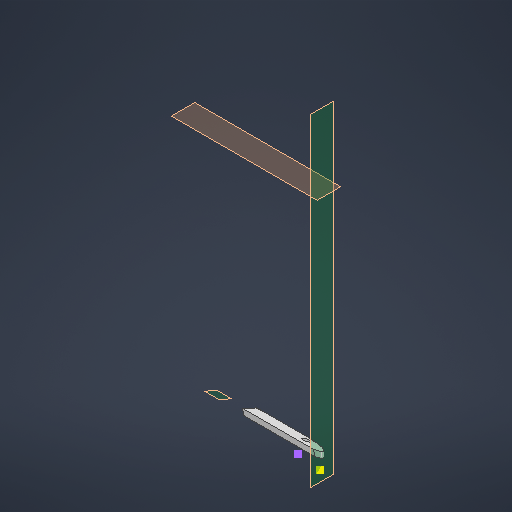
# Autodesk Inventor part: connector
Saved by Autodesk Inventor 2026 (Build 300175050, 175E)
## iProperties
Created: 2026-06-09
Part Number: connector
Material: Generic
Document SubType Name: Modeling
Designer: Delbe
Density: 1 g/cm^3
Appearance: Default
Author: Delbe
Autodesk Inventor part; units mm, degrees
sketch "Sketch5" plane through (0, 0, 0) normal (0, 1, 0) x (-1, 0, 0)
  spline S0 degree 4 poles (214, 0.3449) (213.9235, 0.3586) (213.5504, 0.4255) (212.9247, 0.5375) (211.8694, 0.7251) (210.7617, 0.9209) (209.4043, 1.1592) (207.8102, 1.4368) (205.9789, 1.7525) (203.9169, 2.1042) (201.6282, 2.4897) (199.1185, 2.907) (196.3936, 3.3535) (193.4599, 3.8269) (190.3242, 4.3245) (186.9939, 4.8439) (183.4768, 5.3823) (179.781, 5.937) (175.9152, 6.5054) (171.8885, 7.0847) (167.7102, 7.6721) (163.3902, 8.265) (158.9384, 8.8603) (154.3653, 9.4553) (149.6816, 10.047) (144.8982, 10.6323) (140.0263, 11.2083) (135.0773, 11.7717) (130.0627, 12.3193) (124.9942, 12.8478) (119.8837, 13.3538) (114.7431, 13.8337) (109.5844, 14.2841) (104.4196, 14.7015) (99.2609, 15.0822) (94.1202, 15.4227) (89.0095, 15.7197) (83.9407, 15.9697) (78.9258, 16.1695) (73.9764, 16.3162) (69.104, 16.4071) (64.32, 16.4396) (59.6357, 16.4118) (55.0618, 16.3218) (50.6091, 16.1683) (46.288, 15.9504) (42.1085, 15.6678) (38.0804, 15.3204) (34.213, 14.9088) (30.5154, 14.4338) (26.9962, 13.8969) (23.6634, 13.3) (20.5248, 12.6451) (17.5876, 11.9348) (14.8584, 11.1717) (12.3433, 10.3589) (10.0479, 9.4991) (7.977, 8.5956) (6.1348, 7.651) (4.5247, 6.6676) (3.1496, 5.6471) (2.0123, 4.5896) (1.1163, 3.495) (0.468, 2.3618) (0.0758, 1.1958) (-0.0534, 0) (0.0758, -1.1958) (0.468, -2.3618) (1.1163, -3.495) (2.0123, -4.5896) (3.1496, -5.6471) (4.5247, -6.6676) (6.1348, -7.651) (7.977, -8.5956) (10.0479, -9.4991) (12.3433, -10.3589) (14.8584, -11.1717) (17.5876, -11.9348) (20.5248, -12.6451) (23.6634, -13.3) (26.9962, -13.8969) (30.5154, -14.4338) (34.213, -14.9088) (38.0804, -15.3204) (42.1085, -15.6678) (46.288, -15.9504) (50.6091, -16.1683) (55.0618, -16.3218) (59.6357, -16.4118) (64.32, -16.4396) (69.104, -16.4071) (73.9764, -16.3162) (78.9258, -16.1695) (83.9407, -15.9697) (89.0095, -15.7197) (94.1202, -15.4227) (99.2609, -15.0822) (104.4196, -14.7015) (109.5844, -14.2841) (114.7431, -13.8337) (119.8837, -13.3538) (124.9942, -12.8478) (130.0627, -12.3193) (135.0773, -11.7717) (140.0263, -11.2083) (144.8982, -10.6323) (149.6816, -10.047) (154.3653, -9.4553) (158.9384, -8.8603) (163.3902, -8.265) (167.7102, -7.6721) (171.8885, -7.0847) (175.9152, -6.5054) (179.781, -5.937) (183.4768, -5.3823) (186.9939, -4.8439) (190.3242, -4.3245) (193.4599, -3.8269) (196.3936, -3.3535) (199.1185, -2.907) (201.6282, -2.4897) (203.9169, -2.1042) (205.9789, -1.7525) (207.8102, -1.4368) (209.4043, -1.1592) (210.7617, -0.9209) (211.8694, -0.7251) (212.9247, -0.5375) (213.5504, -0.4255) (213.9235, -0.3586) (214, -0.3449) knots 0 0 0 0 0 0.006275 0.009968 0.014263 0.019074 0.024344 0.030027 0.036088 0.042498 0.04923 0.056263 0.063574 0.071147 0.078961 0.087003 0.095255 0.103702 0.112331 0.121128 0.130079 0.13917 0.148391 0.157726 0.167166 0.176696 0.186306 0.195983 0.205715 0.215491 0.225299 0.235127 0.244964 0.254798 0.264619 0.274414 0.284172 0.293881 0.303532 0.313111 0.322608 0.332012 0.34131 0.350493 0.359549 0.368466 0.377233 0.385838 0.39427 0.402518 0.410569 0.418411 0.426034 0.433424 0.440569 0.447459 0.454083 0.460432 0.466498 0.472281 0.477786 0.483031 0.48805 0.4929 0.497646 0.502354 0.5071 0.51195 0.516969 0.522214 0.527719 0.533502 0.539568 0.545917 0.552541 0.559431 0.566576 0.573966 0.581589 0.589431 0.597482 0.60573 0.614162 0.622767 0.631534 0.640451 0.649507 0.65869 0.667988 0.677392 0.686889 0.696468 0.706119 0.715828 0.725586 0.735381 0.745202 0.755036 0.764873 0.774701 0.784509 0.794285 0.804017 0.813694 0.823304 0.832834 0.842274 0.851609 0.86083 0.869921 0.878872 0.887669 0.896298 0.904745 0.912997 0.921039 0.928853 0.936426 0.943737 0.95077 0.957502 0.963912 0.969973 0.975656 0.980926 0.985737 0.990032 0.993725 1 1 1 1 1
  line L0 (204.525, -2) -> (204.525, 2)
  line L1 (204.525, 0) -> (0, 0)
  line L2 (0, 0) -> (61.2, 0)
  line L3 (61.2, 0) -> (61.2, -16.415)
  line L4 (61.2, -16.415) -> (61.2, 16.415)
  point P0 (0, 0)
  point P1 (213.875, 0.3673)
  point P2 (213.5005, 0.4344)
  point P3 (212.8772, 0.5457)
  point P4 (212.0066, 0.7006)
  point P5 (210.8908, 0.8979)
  point P6 (209.5323, 1.1364)
  point P7 (207.9344, 1.4146)
  point P8 (206.1007, 1.7309)
  point P9 (204.0356, 2.0831)
  point P10 (201.7438, 2.4693)
  point P11 (199.2308, 2.8872)
  point P12 (196.5023, 3.3344)
  point P13 (193.5648, 3.8084)
  point P14 (190.4252, 4.3068)
  point P15 (187.0907, 4.8269)
  point P16 (183.5691, 5.366)
  point P17 (179.8687, 5.9215)
  point P18 (175.9981, 6.4907)
  point P19 (171.9664, 7.0708)
  point P20 (167.7829, 7.6591)
  point P21 (163.4575, 8.2526)
  point P22 (159.0002, 8.8488)
  point P23 (154.4215, 9.4444)
  point P24 (149.732, 10.0368)
  point P25 (144.9427, 10.6228)
  point P26 (140.0648, 11.1993)
  point P27 (135.1097, 11.7633)
  point P28 (130.0889, 12.3114)
  point P29 (125.0142, 12.8402)
  point P30 (119.8974, 13.3464)
  point P31 (114.7505, 13.8266)
  point P32 (109.5855, 14.2771)
  point P33 (104.4145, 14.6943)
  point P34 (99.2495, 15.0749)
  point P35 (94.1026, 15.4151)
  point P36 (88.9858, 15.7116)
  point P37 (83.9111, 15.961)
  point P38 (78.8903, 16.1601)
  point P39 (73.9352, 16.306)
  point P40 (69.0573, 16.3958)
  point P41 (64.268, 16.4271)
  point P42 (59.5785, 16.3978)
  point P43 (54.9998, 16.3062)
  point P44 (50.5425, 16.1509)
  point P45 (46.2171, 15.931)
  point P46 (42.0336, 15.6461)
  point P47 (38.0019, 15.2962)
  point P48 (34.1313, 14.8818)
  point P49 (30.4309, 14.4038)
  point P50 (26.9093, 13.8636)
  point P51 (23.5748, 13.2629)
  point P52 (20.4352, 12.6039)
  point P53 (17.4977, 11.889)
  point P54 (14.7693, 11.1209)
  point P55 (12.2562, 10.3027)
  point P56 (9.9644, 9.4372)
  point P57 (7.8993, 8.5276)
  point P58 (6.0656, 7.5769)
  point P59 (4.4677, 6.5883)
  point P60 (3.1092, 5.5644)
  point P61 (1.9934, 4.5081)
  point P62 (1.1228, 3.4216)
  point P63 (0.4995, 2.307)
  point P64 (0.125, 1.1661)
  point P65 (0.125, -1.1661)
  point P66 (0.4995, -2.307)
  point P67 (1.1228, -3.4216)
  point P68 (1.9934, -4.5081)
  point P69 (3.1092, -5.5644)
  point P70 (4.4677, -6.5883)
  point P71 (6.0656, -7.5769)
  point P72 (7.8993, -8.5276)
  point P73 (9.9644, -9.4372)
  point P74 (12.2562, -10.3027)
  point P75 (14.7693, -11.1209)
  point P76 (17.4977, -11.889)
  point P77 (20.4352, -12.6039)
  point P78 (23.5748, -13.2629)
  point P79 (26.9093, -13.8636)
  point P80 (30.4309, -14.4038)
  point P81 (34.1313, -14.8818)
  point P82 (38.0019, -15.2962)
  point P83 (42.0336, -15.6461)
  point P84 (46.2171, -15.931)
  point P85 (50.5425, -16.1509)
  point P86 (54.9998, -16.3062)
  point P87 (59.5785, -16.3978)
  point P88 (64.268, -16.4271)
  point P89 (69.0573, -16.3958)
  point P90 (73.9352, -16.306)
  point P91 (78.8903, -16.1601)
  point P92 (83.9111, -15.961)
  point P93 (88.9858, -15.7116)
  point P94 (94.1026, -15.4151)
  point P95 (99.2495, -15.0749)
  point P96 (104.4145, -14.6943)
  point P97 (109.5855, -14.2771)
  point P98 (114.7505, -13.8266)
  point P99 (119.8974, -13.3464)
  point P100 (125.0142, -12.8402)
  point P101 (130.0889, -12.3114)
  point P102 (135.1097, -11.7633)
  point P103 (140.0648, -11.1993)
  point P104 (144.9427, -10.6228)
  point P105 (149.732, -10.0368)
  point P106 (154.4215, -9.4444)
  point P107 (159.0002, -8.8488)
  point P108 (163.4575, -8.2526)
  point P109 (167.7829, -7.6591)
  point P110 (171.9664, -7.0708)
  point P111 (175.9981, -6.4907)
  point P112 (179.8687, -5.9215)
  point P113 (183.5691, -5.366)
  point P114 (187.0907, -4.8269)
  point P115 (190.4252, -4.3068)
  point P116 (193.5648, -3.8084)
  point P117 (196.5023, -3.3344)
  point P118 (199.2308, -2.8872)
  point P119 (201.7438, -2.4693)
  point P120 (204.0356, -2.0831)
  point P121 (206.1007, -1.7309)
  point P122 (207.9344, -1.4146)
  point P123 (209.5323, -1.1364)
  point P124 (210.8908, -0.8979)
  point P125 (212.0066, -0.7006)
  point P126 (212.8772, -0.5457)
  point P127 (213.5005, -0.4344)
  point P128 (213.875, -0.3673)
  dimension "d28" = 204.525
  dimension "d29" = 61.2
  dimension "d30" = 32.8299
  constraints: 10 end point, 2 point on line, 1 horizontal, 1 midpoint, 1 perpendicular, 1 vertical, 135 other
  measures "d28" distance of L1.start L1.end
  measures "d29" distance of L1.end L2.end
  measures "d30" distance of L3.end L4.end
extrude "Main Wing" add sketch "Sketch5" along normal blind 453.491
sketch "Sketch6" plane through (-204.525, 0, 2) normal (-1, 0, 0) x (0, 0, 1)
  line L0 (0, 0) -> (0, 66.548)
  line L1 (0, 453.4889) -> (0, 366.5701)
  line L2 (20, 366.5701) -> (-20, 366.5701)
  line L3 (-20, 66.548) -> (20, 66.548)
  line L4 (20, 66.548) -> (20, 366.5701)
  line L5 (-20, 366.5701) -> (-20, 66.548)
  point P0 (-2, 0)
  dimension "d31" = 66.548
  dimension "d32" = 86.9188
  dimension "d33" = 40
  dimension "d34" = 40
  dimension "d43" = 300.0221
  constraints: 12 end point, 3 vertical, 2 horizontal, 2 midpoint
  measures "d31" distance of L0.start L0.end
  measures "d32" distance of L1.start L1.end
  measures "d33" distance of L2.start L2.end
  measures "d34" distance of L3.start L3.end
  measures "d43" distance of L3.end L2.start
extrude "Rectangle Elevron Gap" cut sketch "Sketch6" against normal blind 69.6214
sketch "Sketch7" plane through (-204.525, 66.548, 2) normal (0, 1, 0) x (1, 0, 0)
  line L0 (69.6201, 13.7865) -> (69.6201, -9.7851)
  line L1 (69.6201, -9.7851) -> (69.6201, 2.0009)
  circle A0 centre (69.6201, 2.0009) radius 17
  circle A1 centre (69.6201, 2.0009) radius 1.7526
  point P0 (204.525, 2)
  point P1 (69.6201, 3.7535)
  point P2 (69.6201, 0.2483)
  dimension "d37" = 23.5717
  dimension "d38" = 11.786
  dimension "d41" = 34
  dimension "d42" = 3.5052
  constraints: 4 end point, 2 centre point, 1 coincident, 1 point on line, 1 vertical
  measures "d37" distance of L0.start L0.end
  measures "d38" distance of L0.end L1.end
  measures "d41" diameter of A0
  measures "d42" diameter of A1
extrude "Circle Elevron Gap" cut sketch "Sketch7" along normal blind 300.0221 contours A1 L0 | A0 picked at (69.7501, 0.8471)
sketch "Sketch8" plane through (0, 453.491, 0) normal (0, 1, 0) x (1, 0, 0)
  line L0 (-204.5238, 0) -> (-143.0304, 0)
  circle A0 centre (-143.0304, 0) radius 1.7526
  point P0 (0, 0)
  dimension "d46" = 61.4934
  dimension "d47" = 3.5052
  constraints: 2 end point, 1 centre point, 1 coincident, 1 horizontal
  measures "d46" distance of L0.start L0.end
  measures "d47" diameter of A0
extrude "Elevron Screw Hole" cut sketch "Sketch8" against normal blind 454.0221
ref_plane "Leading Edge Plane" through (0, 226.7455, 0) normal (-1, 0, 0) x (0, 0, 1)
sketch "Sketch9" plane through (0, 226.7455, 0) normal (-1, 0, 0) x (0, 0, 1)
  line L0 (0, -226.7455) -> (0, 226.7401)
  line L1 (0, 226.7401) -> (0, 213.1781)
  line L2 (0, 213.1781) -> (0, 194.4281)
  circle A0 centre (0, 194.4281) radius 18.75
  line L3 (-14.0018, 198.1799) -> (3.7518, 208.4299)
  line L4 (3.7518, 208.4299) -> (14.0018, 190.6764)
  line L5 (14.0018, 190.6764) -> (-3.7518, 180.4264)
  line L6 (-3.7518, 180.4264) -> (-14.0018, 198.1799)
  line L7 (-14.0018, 198.1799) -> (14.0018, 190.6764) construction
  line L8 (3.7518, 208.4299) -> (-3.7518, 180.4264) construction
  circle A1 centre (0, 194.4281) radius 15.5
  dimension "d50" = 13.562
  dimension "d51" = 18.75
  dimension "d52" = 37.5
  dimension "d55" = 20.5
  dimension "d56" = 20.5
  dimension "d70" = 31
  constraints: 18 end point, 2 centre point, 2 coincident, 2 midpoint, 2 parallel, 2 point on line, 1 perpendicular, 1 vertical
  measures "d50" distance of L0.end L1.end
  measures "d51" distance of L1.end L2.end
  measures "d52" diameter of A0
  measures "d55" distance of L4.end L5.end
  measures "d56" distance of L3.end L4.end
  measures "d70" diameter of A1
extrude "Circle thingy for boom" add sketch "Sketch9" along normal blind 204.5 contours A1 L0 L3 L6 L5 | L0 L5 L4 L3 A1 | L5 L6 L3 L0 | L0 L3 L4 L5
sketch "Sketch10" plane through (0, 226.7455, 0) normal (1, 0, 0) x (0, 0, -1)
  line L0 (0, 213.1791) -> (0, 194.4291)
  line L1 (13.6215, 199.3869) -> (-4.9578, 208.0506)
  line L2 (-4.9578, 208.0506) -> (-13.6215, 189.4713)
  line L3 (-13.6215, 189.4713) -> (4.9578, 180.8076)
  line L4 (4.9578, 180.8076) -> (13.6215, 199.3869)
  line L5 (13.6215, 199.3869) -> (-13.6215, 189.4713) construction
  line L6 (-4.9578, 208.0506) -> (4.9578, 180.8076) construction
  point P0 (0, -226.7455)
  dimension "d57" = 18.75
  dimension "d58" = 20.5
  dimension "d59" = 20.5
  constraints: 14 end point, 2 parallel, 1 perpendicular, 1 vertical
  measures "d57" distance of L0.start L0.end
  measures "d58" distance of L3.end L2.end
  measures "d59" distance of L2.end L1.end
extrude "20x20 hole for boom" cut sketch "Sketch10" against normal blind 205.5
ref_plane "Plane of Pain" through (-204.525, 0, -17) normal (0, 0, 1) x (0, 1, 0)
ref_plane "Work Plane5" through (-204.525, 0, -2) normal (0, 0, 1) x (0, 1, 0)
sketch "Sketch11" plane through (-204.525, 0, -17) normal (0, 0, 1) x (0, 1, 0)
  line L0 (453.4842, 0.0013) -> (403.4842, 0.0013)
  line L1 (403.4842, 0.0013) -> (404.7122, -149.9936)
  circle A0 centre (404.7122, -149.9936) radius 5.25
  line L2 (404.7122, -149.9936) -> (219.7122, -149.9936)
  circle A1 centre (219.7122, -149.9936) radius 5.25
  line L3 (366.5707, -80.63) -> (219.7122, -80.63)
  line L4 (219.7122, -80.63) -> (219.7122, -149.9936)
  point P0 (0, -204.525)
  dimension "d64" = 50
  dimension "d65" = 150
  dimension "d66" = 10.5
  dimension "d67" = 185
  dimension "d121" = 146.8585
  dimension "d122" = 69.3637
  constraints: 10 end point, 3 horizontal, 2 centre point, 2 coincident, 1 equal radius, 1 perpendicular
  measures "d64" distance of L0.start L0.end
  measures "d65" distance of L0.end L1.end
  measures "d66" diameter of A0
  measures "d67" distance of L2.start L2.end
  measures "d121" distance of L3.start L3.end
  measures "d122" distance of L3.end L4.end
ref_plane "20x20 Plane" through (0, 416.8428, -9.2897) normal (0, 0.4226183, 0.9063078) x (1, 0, 0)
sketch "Sketch12" plane through (0, 416.8428, -9.2897) normal (0, 0.4226183, 0.9063078) x (1, 0, 0)
  line L0 (0, 10.2503) -> (0, 0.0003)
  line L1 (0, 0.0003) -> (-55, 0.0003)
  circle A0 centre (-55, 0.0003) radius 5.25
  circle A1 centre (-55, 0.0003) radius 2.75
  point P0 (0, -381.7138)
  dimension "d71" = 10.25
  dimension "d72" = 55
  dimension "d73" = 10.5
  dimension "d74" = 5.5
  constraints: 4 end point, 3 coincident, 2 centre point, 1 horizontal, 1 vertical
  measures "d71" distance of L0.start L0.end
  measures "d72" distance of L0.end L1.end
  measures "d73" diameter of A0
  measures "d74" diameter of A1
sketch "Sketch13" plane through (0, 416.8428, -9.2897) normal (0, 0.4226183, 0.9063078) x (1, 0, 0)
  circle A0 centre (-55, 0) radius 5.25
  circle A1 centre (-55, 0) radius 2.75
  point P0 (0, -381.7138)
  dimension "d77" = 10.5
  dimension "d82" = 5.5
  constraints: 2 centre point, 1 coincident
  measures "d77" diameter of A0
  measures "d82" diameter of A1
extrude "Boom Screw Head" cut sketch "Sketch13" against normal blind 13.75 contours A0 | A1
extrude "Boom Screw Hole" add sketch "Sketch12" against normal blind 3
sketch "Sketch14" plane through (-204.525, 366.5701, -2) normal (0, -1, 0) x (1, 0, 0)
  line L0 (61.5404, 3.7631) -> (61.5404, 7.2141)
  line L1 (61.5404, 7.2141) -> (43.5474, 7.2141)
  line L2 (61.5404, 7.2141) -> (69.3184, 7.2141)
  line L3 (43.5474, 7.2141) -> (43.5474, -10.2859)
  line L4 (69.3184, 7.2141) -> (69.3184, -10.2859)
  line L5 (43.5474, -10.2859) -> (69.3184, -10.2859)
  point P0 (204.525, 2)
  dimension "d89" = 3.451
  dimension "d90" = 17.993
  dimension "d91" = 7.778
  dimension "d93" = 17.5
  dimension "d94" = 17.5
  constraints: 12 end point, 3 vertical, 2 horizontal
  measures "d89" distance of L0.start L0.end
  measures "d90" distance of L0.end L1.end
  measures "d91" distance of L0.end L2.end
  measures "d93" distance of L1.end L3.end
  measures "d94" distance of L2.end L4.end
extrude "Servo Hole" cut sketch "Sketch14" against normal blind 28.763
sketch "Sketch15" plane through (-135.2066, 366.5701, -11.7525) normal (-1, 0, 0) x (0, 0, 1)
  line L0 (17, 0) -> (17, 6)
  line L1 (17, 6) -> (17, 8)
  line L2 (17, 8) -> (-3, 8)
  line L3 (-3, 8) -> (-3, 6)
  line L4 (-3, 6) -> (17, 6)
  point P0 (11.7525, -366.5701)
  dimension "d97" = 6
  dimension "d98" = 2
  dimension "d99" = 2
  constraints: 10 end point, 2 perpendicular, 1 point on line, 1 vertical
  measures "d97" distance of L0.start L0.end
  measures "d98" distance of L0.end L1.end
  measures "d99" distance of L2.end L3.end
extrude "Servo Sidewall 1" cut sketch "Sketch15" against normal blind 2.782
sketch "Sketch16" plane through (-160.9776, 366.5701, 5.2141) normal (1, 0, 0) x (0, 0, -1)
  line L0 (0, 0) -> (0, 6)
  line L1 (0, 6) -> (0, 8)
  line L2 (0, 8) -> (14, 8)
  line L3 (14, 8) -> (14, 6)
  line L4 (14, 6) -> (0, 6)
  point P0 (5.2141, -366.5701)
  dimension "d102" = 6
  dimension "d103" = 2
  constraints: 10 end point, 2 perpendicular, 1 point on line, 1 vertical
  measures "d102" distance of L0.start L0.end
  measures "d103" distance of L0.end L1.end
extrude "Servo Sidewall 2" cut sketch "Sketch16" against normal blind 2.782
sketch "Sketch17" plane through (-135.2066, 366.5701, 5.2141) normal (0, 0, -1) x (-1, 0, 0)
  line L0 (0, 8) -> (0, 16.3)
  line L1 (0, 28.7478) -> (0, 23.2698)
  line L2 (0, 16.3) -> (-27.1565, 48.6638)
  line L3 (0, 23.2698) -> (-27.1565, 55.6336)
  line L4 (-27.1565, 48.6638) -> (-27.1565, 55.6336)
  line L5 (0, 23.2698) -> (0, 16.3)
  point P0 (-135.2066, -366.5701)
  point P1 (0, 23.2698)
  dimension "d106" = 8.3
  dimension "d107" = 5.478
  dimension "d108" = 42.248
  dimension "d109" = 42.248
  constraints: 12 end point, 3 vertical, 1 coincident, 1 point on line
  measures "d106" distance of L0.end L0.start
  measures "d107" distance of L1.end L1.start
  measures "d108" distance of L2.start L2.end
  measures "d109" distance of L3.start L3.end
extrude "some slant hole" cut sketch "Sketch17" along normal blind 23.75
fillet "Fillet for slant" radius 7.7 2 edges at (-135.2066, 382.8701, -3.2692) (-135.2066, 389.8399, -3.2692)
sketch "Sketch18" plane through (-204.525, 0, -17) normal (0, 0, 1) x (0, 1, 0)
  circle A0 centre (219.7124, -149.9979) radius 3.25
  point P0 (0, -204.525)
  dimension "d113" = 6.5
  constraints: 1 centre point
  measures "d113" diameter of A0
extrude "Screwhead for something" cut sketch "Sketch11" along normal blind 5.25 contours A1 L4 L2 | L2 L4 A1
extrude "screwhole for thingy" cut sketch "Sketch18" along normal blind 41.75
ref_plane "Work Plane10" through (-182.7513, 87.2769, 166.4641) normal (0, 0.8660254, -0.5) x (1, 0, 0)
ref_plane "Work Plane9" through (-182.7513, 366.5701, 5.2141) normal (0, 0.8660254, -0.5) x (1, 0, 0)
sketch "Sketch20" plane through (-182.7513, 87.2769, 166.4641) normal (0, 0.8660254, -0.5) x (1, 0, 0)
  circle A0 centre (138, 200) radius 2.8284
  point P0 (182.7513, 187.8006)
  constraints: 1 centre point
ref_plane "Bottom of Airfoil" through (-204.525, 0, 16.5) normal (0, 0, 1) x (0, 1, 0)
sketch "Sketch21" plane through (-204.525, 0, 16.5) normal (0, 0, 1) x (0, 1, 0)
  line L0 (366.5707, -80.6294) -> (219.7127, -80.6294)
  line L1 (219.7127, -80.6294) -> (219.7127, -149.9934)
  line L2 (219.7127, -149.9934) -> (214.6627, -149.9934)
  line L3 (214.6627, -147.0779) -> (214.6627, -152.9089)
  line L4 (214.6627, -147.0779) -> (219.7125, -144.1624)
  line L5 (219.7125, -144.1624) -> (224.7623, -147.0779)
  line L6 (224.7623, -147.0779) -> (224.7623, -152.9089)
  line L7 (224.7623, -152.9089) -> (219.7125, -155.8244)
  line L8 (214.6627, -152.9089) -> (219.7125, -155.8244)
  point P0 (0, -204.525)
  point P1 (224.7623, -147.0779)
  dimension "d123" = 146.858
  dimension "d124" = 69.364
  dimension "d125" = 5.05
  dimension "d126" = 5.831
  dimension "d127" = 5.831
  dimension "d128" = 5.831
  dimension "d129" = 5.831
  dimension "d130" = 5.831
  constraints: 18 end point, 2 perpendicular, 1 horizontal, 1 midpoint, 1 vertical
  measures "d123" distance of L0.start L0.end
  measures "d124" distance of L0.end L1.end
  measures "d125" distance of L1.end L2.end
  measures "d126" distance of L3.start L3.end
  measures "d127" distance of L4.end L4.start
  measures "d128" distance of L5.end L5.start
  measures "d129" distance of L6.end L6.start
  measures "d130" distance of L7.start L7.end
extrude "Hexagon Hole of Doom" cut sketch "Sketch21" against normal blind 4
sketch "Sketch22" plane through (-182.7513, 87.2769, 166.4641) normal (0, 0.8660254, -0.5) x (1, 0, 0)
  line L0 (138, 200) -> (153, 200)
  line L1 (153, 200) -> (153, 185)
  circle A0 centre (153, 185) radius 5.25
  line L2 (153, 185) -> (61.5, 185)
  circle A1 centre (61.5, 185) radius 5.25
  point P0 (182.7513, 187.8006)
  dimension "d137" = 15
  dimension "d138" = 15
  dimension "d139" = 10.5
  dimension "d140" = 91.5
  dimension "d141" = 10.5
  constraints: 6 end point, 2 centre point, 2 coincident, 2 horizontal, 1 vertical
  measures "d137" distance of L0.start L0.end
  measures "d138" distance of L0.end L1.end
  measures "d139" diameter of A0
  measures "d140" distance of L2.start L2.end
  measures "d141" diameter of A1
extrude "Extrusion23" cut sketch "Sketch22" along normal blind 68.25
sketch "Sketch23" plane through (-182.7513, 87.2769, 166.4641) normal (0, 0.8660254, -0.5) x (1, 0, 0)
  line L0 (138, 200) -> (153, 200)
  line L1 (153, 200) -> (153, 185)
  line L2 (153, 185) -> (61.5, 185)
  circle A0 centre (153, 185) radius 5.25
  circle A1 centre (153, 185) radius 3.25
  circle A2 centre (61.5, 185) radius 5.25
  circle A3 centre (61.5, 185) radius 3.25
  point P0 (182.7513, 187.8006)
  dimension "d144" = 15
  dimension "d145" = 15
  dimension "d146" = 91.5
  dimension "d147" = 10.5
  dimension "d148" = 6.5
  dimension "d149" = 10.5
  dimension "d150" = 6.5
  constraints: 6 end point, 4 centre point, 4 coincident, 2 perpendicular, 1 horizontal
  measures "d144" distance of L0.start L0.end
  measures "d145" distance of L0.end L1.end
  measures "d146" distance of L1.end L2.end
  measures "d147" diameter of A0
  measures "d148" diameter of A1
  measures "d149" diameter of A2
  measures "d150" diameter of A3
extrude "Extrusion24" add sketch "Sketch23" along normal blind 20 contours A0 L2 A1 L1 | L1 A1 L2 A0 | A2
sketch "Sketch24" plane through (0, 0, 0) normal (0, -1, 0) x (1, 0, 0)
  line L0 (0, -15) -> (-205, -15)
  line L1 (-205, -15) -> (-205, 16)
  line L2 (-205, 16) -> (0, 16)
  line L3 (0, 16) -> (0, -15)
  point P0 (0, 0)
  constraints: 8 end point, 2 parallel, 1 horizontal, 1 perpendicular
extrude "Extrusion25" cut sketch "Sketch24" along normal blind 8.75
sketch "Sketch25" plane through (0, 226.7455, 0) normal (-1, 0, 0) x (0, 0, 1)
  line L0 (-16.4393, -226.7455) -> (20.5607, -226.7455) construction
  line L1 (17.0941, -211.1086) -> (17.0941, -226.7455)
  line L2 (17.0941, -226.7455) -> (-16.4393, -226.7455)
  line L3 (-16.4393, -226.7455) -> (36.2607, -226.7455) construction
  line L4 (-16.4393, -226.7455) -> (17.4356, -226.7455)
  line L5 (0, -226.7455) -> (0, -219.0797)
  line L6 (17.0941, -201.9506) -> (17.0941, -211.1086)
  line L7 (-36.0788, -226.7455) -> (-16.4393, -226.7455)
  line L8 (-6.752, -213.0525) -> (6.5452, -213.0525) construction
  line L9 (-6.752, -222.2282) -> (6.752, -215.9312)
  line L10 (6.752, -215.9312) -> (7.5873, -206.3837)
  line L11 (7.5873, -206.3837) -> (-14.6028, -216.7311)
  line L12 (-14.6028, -216.7311) -> (-6.752, -222.2282)
  line L13 (-16.4393, -226.7455) -> (17.0941, -211.1086)
  line L14 (17.0941, -226.7455) -> (-16.4393, -226.7455)
  line L15 (-16.4393, -226.7455) -> (-16.4393, 228)
  line L16 (-16.4393, 228) -> (17.0941, 228)
  line L17 (17.0941, 228) -> (17.0941, -226.7455)
  dimension "d155" = 37
  dimension "d220" = 14.9
  dimension "d221" = 60
  dimension "d222" = 60
  dimension "d223" = 8.3
  constraints: 36 end point, 5 horizontal, 3 parallel, 3 vertical, 2 perpendicular, 1 collinear, 1 midpoint, 1 point on line
  measures "d155" distance of L0.start L1.start
  measures "d220" distance of L9.start L9.end
  measures "d221" angle of L10 L11
  measures "d222" angle of L12 L11
  measures "d223" distance between parallel lines of L9 L11
ref_plane "Work Plane14" through (0, 366.491, 0) normal (0, 1, 0) x (1, 0, 0)
ref_plane "Work Plane15" through (-168.2987, 4.1455, -7.5873) normal (0, -0.9063078, 0.4226183) x (1, 0, 0)
extrude "Extrusion36" cut sketch "Sketch25" along normal blind 236.5 contours L13 L10 L11 L12 L15 L16 L17 L6 | L1 L2 L5 L9 L13 | L2 L13 L9 L5
sketch "Sketch35" plane through (-174.1935, 4.5173, -6.752) normal (0, -0.9063078, 0.4226183) x (1, 0, 0)
  line L0 (174.1935, 4.2103) -> (59.1935, 4.2103)
  line L1 (59.1935, 4.2103) -> (59.1935, 22)
  line L2 (59.1935, 22) -> (-35, 22)
  line L3 (-35, 22) -> (-35, -11)
  line L4 (-35, -11) -> (59.1935, -11)
  line L5 (59.1935, -11) -> (59.1935, 4.2103)
  dimension "d226" = 115
  constraints: 12 end point, 5 perpendicular, 1 horizontal, 1 point on line
  measures "d226" distance of L0.start L0.end
extrude "Extrusion37" cut sketch "Sketch35" against normal blind 236.5
ref_plane "Work Plane8" through (0, 0, 0) normal (0, -1, 0) x (1, 0, 0)
body "Solid3"
